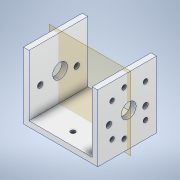
# Autodesk Inventor part: hand1
Saved by Autodesk Inventor 2022 (Build 260153000, 153)
## iProperties
Created: 2022-04-20
Part Number: hand1
Material: アルミニウム 6061
Document SubType Name: Modeling
Designer: Yazawa
Density: 2.7 g/cm^3
Appearance: アルミニウム - フラット
Author: Yazawa
Autodesk Inventor part; units mm, degrees
ref_plane "YZ Plane" through (0, 0, 0) normal (1, 0, 0) x (0, 1, 0)
ref_plane "XZ Plane" through (0, 0, 0) normal (0, 1, 0) x (-1, 0, 0)
ref_plane "XY Plane" through (0, 0, 0) normal (0, 0, 1) x (1, 0, 0)
sketch "スケッチ1" plane through (0, 0, 0) normal (0, 1, 0) x (-1, 0, 0)
  line L0 (20, -20) -> (-20, -20)
  line L1 (-20, -20) -> (-20, 20)
  line L2 (-20, 20) -> (20, 20)
  line L3 (20, 20) -> (20, -20)
  line L4 (-20, 20) -> (20, -20) construction
  line L5 (-20, -20) -> (20, 20) construction
  point P0 (0, 0)
  point P1 (0, 0)
  dimension "d0" = 40
  dimension "d1" = 40
  constraints: 12 end point, 2 midpoint, 2 parallel, 1 coincident, 1 horizontal, 1 perpendicular
  measures "d0" distance of L1.end L2.end
  measures "d1" distance of L0.end L1.end
extrude "押し出し1" add sketch "スケッチ1" along normal blind 3
sketch "スケッチ2" plane through (0, 3, 0) normal (0, 1, 0) x (1, 0, 0)
  line L0 (-20, -20) -> (20, -20) projected
  line L1 (20, -20) -> (20, 20) projected
  line L2 (20, 20) -> (-20, 20) projected
  line L3 (-20, 20) -> (-20, -20) projected
  line L4 (-20, -20) -> (20, -20) projected
  line L5 (-20, -20) -> (-17, -20)
  line L6 (-17, -20) -> (-17, 20)
  line L7 (-17, 20) -> (-20, 20)
  line L8 (-20, 20) -> (-20, -20)
  line L9 (20, -20) -> (20, 20) projected
  line L10 (20, -20) -> (17, -20)
  line L11 (17, -20) -> (17, 20)
  line L12 (17, 20) -> (20, 20)
  line L13 (20, 20) -> (20, -20)
  line L14 (20, 20) -> (-20, 20) projected
  point P0 (0, 0)
  point P1 (-17, 20)
  dimension "d4" = 3
  dimension "d5" = 3
  constraints: 16 end point, 4 parallel, 2 collinear, 2 horizontal, 2 perpendicular
  measures "d4" distance of L7.end L6.end
  measures "d5" distance of L11.end L12.end
extrude "押し出し2" add sketch "スケッチ2" along normal blind 40 from surface at -3 contours L3 L2 L6 L0 | L11 L2 L1 L0
sketch "スケッチ3" plane through (20, 0, 20) normal (1, 0, 0) x (0, 0, -1)
  line L0 (0, 3) -> (40, 3) projected
  line L1 (25, 18) -> (40, 18) construction
  line L2 (40, 40) -> (40, 3) construction
  line L3 (25, 18) -> (-0.0782, 18) construction
  point P0 (20, 0)
  dimension "d8" = 15
  dimension "d50" = 15
  constraints: 4 end point, 2 point on line, 1 horizontal
  measures "d8" distance from line of L0 L1.start
  measures "d50" distance of L1.start L1.end
hole "穴1" at (20, 18, -5) direction (-1, 0, 0) diameter 8 end through all
sketch "スケッチ5" plane through (20, 0, 20) normal (1, 0, 0) x (0, 0, -1)
  line L0 (0, 0) -> (0, 40) projected
  line L1 (0, 0) -> (40, 0) projected
  line L2 (40, 33) -> (10, 33)
  line L3 (10, 33) -> (10, 3)
  line L4 (10, 3) -> (40, 3)
  line L5 (40, 3) -> (40, 33)
  line L6 (40, 33) -> (10, 3) construction
  line L7 (40, 3) -> (10, 33) construction
  line L8 (40, 18) -> (10, 18)
  circle A0 centre (25, 18) radius 4 projected
  point P0 (20, 0)
  point P1 (34, 27)
  point P2 (16, 27)
  point P3 (16, 9)
  point P4 (34, 9)
  point P5 (34, 27)
  dimension "d20" = 30
  dimension "d21" = 30
  dimension "d23" = 6
  dimension "d24" = 6
  dimension "d27" = 360
  dimension "d40" = 0
  constraints: 14 end point, 4 coincident, 3 midpoint, 2 parallel, 1 horizontal, 1 perpendicular, 1 symmetric about line, 7 other
  measures "d20" distance of L4.end L3.end
  measures "d21" distance of L3.end L2.end
  measures "d23" distance from line of L5 point (34, 27)
  measures "d24" distance from line of L2 point (34, 27)
  measures "d40" distance of point (25, 18) point (25, 18)
hole "穴2" at (20, 27, -14) at (20, 9, -14) at (20, 27, 4) at (20, 9, 4) direction (-1, 0, 0) diameter 2.459 depth 3 thread size "M3x0.5" class "6H" standard "ISO Metric profile"
sketch "スケッチ6" plane through (0, 3, 0) normal (0, 1, 0) x (1, 0, 0)
  line L0 (17, 20) -> (-17, 20) projected
  point P0 (0, 0)
  point P1 (0, 15)
  point P2 (0, -5)
  point P3 (0, 20)
  dimension "d41" = 5
  dimension "d42" = 20
  constraints: 2 vertical alignment, 1 midpoint
  measures "d41" distance from line of L0 point (0, 15)
  measures "d42" distance of point (0, -5) point (0, 15)
hole "穴3" at (0, 3, -15) at (0, 3, 5) direction (0, -1, 0) diameter 2.459 depth 3 thread size "M3x0.5" class "6H" standard "ISO Metric profile"
sketch "スケッチ8" plane through (20, 0, 20) normal (1, 0, 0) x (0, 0, -1)
  circle A0 centre (25, 18) radius 4 projected
  line L0 (22.5, 30) -> (22.5, 6) construction
  point P0 (20, 0)
  dimension "d56" = 24
  dimension "d57" = 12
  dimension "d58" = 2.5
  constraints: 2 coincident, 2 end point, 1 vertical
  measures "d56" distance of L0.start L0.end
  measures "d57" vertical distance of A0.centre L0.start
  measures "d58" distance from line of L0 A0.centre
hole "穴4" at (20, 30, -2.5) at (20, 6, -2.5) direction (-1, 0, 0) diameter 2.459 depth 3 tip angle 118 thread size "M3x0.5" class "6H" standard "ISO Metric profile"
sketch "スケッチ9" plane through (20, 0, 20) normal (1, 0, 0) x (0, 0, -1)
  circle A0 centre (25, 18) radius 4 projected
  line L0 (0, 18) -> (25, 18)
  line L1 (0, 0) -> (0, 40) projected
  line L2 (40, 0) -> (40, 40) projected
  line L3 (25, 18) -> (4.9598, 29.5702)
  line L4 (25, 18) -> (43.9658, 28.9499)
  circle A1 centre (14.3, 16.6721) radius 1.5
  circle A2 centre (34, 15.6906) radius 1.5
  line L5 (22.5, 13.6699) -> (4.2655, 24.1976)
  line L6 (27.5, 13.6699) -> (35.6852, 18.3956)
  point P0 (20, 0)
  dimension "d70" = 3
  dimension "d71" = 3
  dimension "d72" = 14.3
  dimension "d73" = 6
  dimension "d83" = 5
  dimension "d84" = 5
  dimension "d85" = 30
  dimension "d86" = 30
  constraints: 11 end point, 2 centre point, 2 coincident, 2 parallel, 2 tangent, 1 horizontal, 1 point on line
  measures "d70" diameter of A2
  measures "d71" diameter of A1
  measures "d72" distance from line of L1 A1.centre
  measures "d73" distance from line of L2 A2.centre
  measures "d83" distance between parallel lines of L3 L5
  measures "d84" distance between parallel lines of L4 L6
  measures "d85" angle of L3 L0
  measures "d86" angle of L4 L0
hole "穴5" at (20, 16.6721, 5.7) at (20, 15.6906, -14) direction (-1, 0, 0) diameter 3 depth 40
ref_plane "作業平面1" through (0, 3, 20) normal (1, 0, 0) x (0, 0, -1)
sketch "スケッチ11" plane through (0, 0, 0) normal (0, -1, 0) x (1, 0, 0)
  line L0 (20, -20) -> (20, 20) projected
  line L1 (20, -20) -> (-20, -20)
  line L2 (-20, -20) -> (-20, 11.7)
  line L3 (-20, 11.7) -> (20, 11.7)
  line L4 (20, 11.7) -> (20, -20)
  line L5 (-20, -20) -> (-20, 20) projected
  point P0 (0, 0)
  dimension "d87" = 31.7
  constraints: 8 end point, 2 parallel, 1 collinear, 1 horizontal, 1 perpendicular
  measures "d87" distance of L1.end L2.end
extrude "押し出し5" cut sketch "スケッチ11" against normal blind 35.85 keep common part
ref_plane "作業平面2" through (-20, 0, -4.15) normal (0, 0, 1) x (1, 0, 0)
